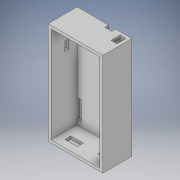
# Autodesk Inventor part: Smart Lock Box Bottom Correct
Saved by Autodesk Inventor 2019.3 (Build 233278000, 278)
## iProperties
Created: 2019-04-11
Part Number: Smart Lock Box Bottom Correct
Material: Generic
Document SubType Name: Modeling
Designer: grego
Density: 1 g/cm^3
Appearance: Default
Author: grego
Autodesk Inventor part; units mm, degrees
ref_plane "YZ Plane" through (0, 0, 0) normal (1, 0, 0) x (0, 1, 0)
ref_plane "XZ Plane" through (0, 0, 0) normal (0, 1, 0) x (-1, 0, 0)
ref_plane "XY Plane" through (0, 0, 0) normal (0, 0, 1) x (1, 0, 0)
sketch "Sketch1" plane through (0, 0, 0) normal (0, 0, 1) x (1, 0, 0)
  line L0 (-50.7629, 56.7485) -> (-50.7629, -66.1875)
  line L1 (-50.7629, -66.1875) -> (15.2771, -66.1875)
  line L2 (15.2771, -66.1875) -> (15.2771, 56.7485)
  line L3 (15.2771, 56.7485) -> (-50.7629, 56.7485)
  point P0 (0, 0)
  dimension "d0" = 122.936
  dimension "d1" = 66.04
  constraints: 8 end point, 3 perpendicular, 1 vertical
  measures "d0" distance between parallel lines of L1 L3
  measures "d1" distance between parallel lines of L2 L0
extrude "Extrusion1" add sketch "Sketch1" along normal blind 35.052
sketch "Sketch2" plane through (0, 0, 35.052) normal (0, 0, 1) x (1, 0, 0)
  line L0 (-47.2069, 53.1925) -> (11.7211, 53.1925)
  line L1 (11.7211, 53.1925) -> (11.7211, -62.6315)
  line L2 (11.7211, -62.6315) -> (-47.2069, -62.6315)
  line L3 (-47.2069, -62.6315) -> (-47.2069, 53.1925)
  line L4 (15.2771, 56.7485) -> (-50.7629, 56.7485) projected
  line L5 (15.2771, -66.1875) -> (15.2771, 56.7485) projected
  line L6 (-50.7629, -66.1875) -> (15.2771, -66.1875) projected
  line L7 (-50.7629, 56.7485) -> (-50.7629, -66.1875) projected
  point P0 (0, 0)
  dimension "d4" = 3.556
  dimension "d5" = 3.556
  dimension "d6" = 3.556
  dimension "d7" = 3.556
  constraints: 8 end point, 2 parallel, 1 horizontal, 1 perpendicular
  measures "d4" distance between parallel lines of L0 L4
  measures "d5" distance between parallel lines of L5 L1
  measures "d6" distance between parallel lines of L6 L2
  measures "d7" distance between parallel lines of L7 L3
extrude "Extrusion2" cut sketch "Sketch2" against normal blind 31.5 contours L0 L1 L2 L3
sketch "Sketch3" plane through (-50.7629, -66.1875, 0) normal (0, -1, 0) x (1, 0, 0)
  line L0 (11.556, 26.552) -> (26.556, 26.552)
  line L1 (26.556, 26.552) -> (26.556, 19.052)
  line L2 (26.556, 19.052) -> (11.556, 19.052)
  line L3 (11.556, 19.052) -> (11.556, 26.552)
  line L4 (62.484, 3.552) -> (3.556, 3.552) projected
  line L5 (3.556, 35.052) -> (3.556, 3.552) projected
  line L6 (46.484, 21.552) -> (56.484, 21.552)
  line L7 (56.484, 21.552) -> (56.484, 16.552)
  line L8 (56.484, 16.552) -> (46.484, 16.552)
  line L9 (46.484, 16.552) -> (46.484, 21.552)
  line L10 (62.484, 35.052) -> (62.484, 3.552) projected
  point P0 (50.7629, 0)
  dimension "d10" = 23
  dimension "d11" = 8
  dimension "d12" = 7.5
  dimension "d13" = 15
  dimension "d14" = 18
  dimension "d15" = 5
  dimension "d16" = 10
  dimension "d17" = 16
  constraints: 16 end point, 4 parallel, 2 horizontal, 2 perpendicular
  measures "d10" distance between parallel lines of L4 L0
  measures "d11" distance between parallel lines of L5 L3
  measures "d12" distance between parallel lines of L2 L0
  measures "d13" distance between parallel lines of L1 L3
  measures "d14" distance between parallel lines of L4 L6
  measures "d15" distance between parallel lines of L8 L6
  measures "d16" distance between parallel lines of L7 L9
  measures "d17" distance between parallel lines of L10 L9
extrude "Extrusion3" cut sketch "Sketch3" against normal blind 3.56
sketch "Sketch4" plane through (0, 0, 0) normal (0, 0, -1) x (-1, 0, 0)
  line L0 (42.1269, -34.1315) -> (47.2069, -34.1315)
  line L1 (47.2069, -34.1315) -> (47.2069, -57.1315)
  line L2 (47.2069, -57.1315) -> (42.1269, -57.1315)
  line L3 (42.1269, -57.1315) -> (42.1269, -34.1315)
  line L4 (47.2069, -62.6315) -> (47.2069, 53.1925) projected
  line L5 (-11.7211, -62.6315) -> (47.2069, -62.6315) projected
  line L6 (40.2069, 30.1925) -> (47.2069, 30.1925)
  line L7 (47.2069, 30.1925) -> (47.2069, 23.1925)
  line L8 (47.2069, 23.1925) -> (40.2069, 23.1925)
  line L9 (40.2069, 23.1925) -> (40.2069, 30.1925)
  line L10 (47.2069, 53.1925) -> (-11.7211, 53.1925) projected
  line L11 (4.2789, 53.1925) -> (12.7789, 53.1925)
  line L12 (12.7789, 53.1925) -> (12.7789, 44.1925)
  line L13 (12.7789, 44.1925) -> (4.2789, 44.1925)
  line L14 (4.2789, 44.1925) -> (4.2789, 53.1925)
  line L15 (-11.7211, 53.1925) -> (-11.7211, -62.6315) projected
  point P0 (0, 0)
  dimension "d20" = 0
  dimension "d21" = 5.5
  dimension "d22" = 23
  dimension "d23" = 5.08
  dimension "d24" = 30
  dimension "d25" = 7
  dimension "d26" = 7
  dimension "d27" = 0
  dimension "d28" = 9
  dimension "d29" = 8.5
  dimension "d30" = 0
  dimension "d31" = 16
  constraints: 24 end point, 6 parallel, 3 horizontal, 3 perpendicular
  measures "d20" distance between parallel lines of L4 L1
  measures "d21" distance between parallel lines of L5 L2
  measures "d22" distance between parallel lines of L2 L0
  measures "d23" distance between parallel lines of L1 L3
  measures "d24" distance between parallel lines of L10 L8
  measures "d25" distance between parallel lines of L8 L6
  measures "d26" distance between parallel lines of L7 L9
  measures "d27" distance between parallel lines of L4 L7
  measures "d28" distance between parallel lines of L13 L11
  measures "d29" distance between parallel lines of L12 L14
  measures "d30" distance between parallel lines of L10 L11
  measures "d31" distance between parallel lines of L14 L15
extrude "Extrusion4" cut sketch "Sketch4" against normal blind 3.56 contours L0 L1 L2 L3 | L8 L9 L6 L4 | L12 L13 L14 L10
sketch "Sketch5" plane through (-50.7629, 56.7485, 0) normal (0, 1, 0) x (1, 0, 0)
  line L0 (62.484, -14.552) -> (55.484, -14.552)
  line L1 (55.484, -14.552) -> (55.484, -3.552)
  line L2 (55.484, -3.552) -> (62.484, -3.552)
  line L3 (62.484, -3.552) -> (62.484, -14.552)
  line L4 (62.484, -35.052) -> (62.484, -3.552) projected
  line L5 (46.484, -3.552) -> (62.484, -3.552) projected
  line L6 (46.484, -4.552) -> (37.984, -4.552)
  line L7 (37.984, -4.552) -> (37.984, 2.448)
  line L8 (37.984, 2.448) -> (46.484, 2.448)
  line L9 (46.484, 2.448) -> (46.484, -4.552)
  line L10 (46.484, -3.552) -> (37.984, -3.552) projected
  point P0 (50.7629, 0)
  dimension "d34" = 11
  dimension "d35" = 0
  dimension "d37" = 7
  dimension "d39" = 16
  dimension "d40" = 7
  dimension "d41" = 8.5
  dimension "d50" = 1
  constraints: 16 end point, 4 parallel, 2 horizontal, 2 perpendicular
  measures "d34" distance between parallel lines of L2 L0
  measures "d35" distance between parallel lines of L4 L3
  measures "d37" distance between parallel lines of L1 L3
  measures "d39" distance between parallel lines of L3 L9
  measures "d40" distance between parallel lines of L8 L6
  measures "d41" distance between parallel lines of L7 L9
  measures "d50" distance between parallel lines of L6 L10
extrude "Extrusion5" cut sketch "Sketch5" against normal blind 3.56
sketch "Sketch6" plane through (-50.7629, -66.1875, 0) normal (-1, 0, 0) x (0, 0, 1)
  line L0 (13.552, 98.38) -> (18.552, 98.38)
  line L1 (18.552, 98.38) -> (18.552, 87.38)
  line L2 (18.552, 87.38) -> (13.552, 87.38)
  line L3 (13.552, 87.38) -> (13.552, 98.38)
  line L4 (3.552, 122.936) -> (3.552, 3.556) projected
  line L5 (35.052, 119.38) -> (3.552, 119.38) projected
  point P0 (0, 66.1875)
  dimension "d44" = 15
  dimension "d45" = 5
  dimension "d46" = 11
  dimension "d47" = 32
  constraints: 8 end point, 2 parallel, 1 horizontal, 1 perpendicular
  measures "d44" distance between parallel lines of L4 L1
  measures "d45" distance between parallel lines of L1 L3
  measures "d46" distance between parallel lines of L2 L0
  measures "d47" distance between parallel lines of L5 L2
extrude "Extrusion6" cut sketch "Sketch6" against normal blind 3.56
body "Solid1"
